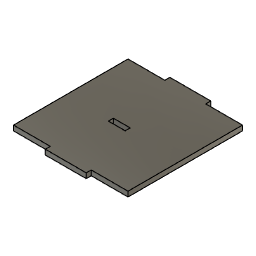
ProjectMiddle (Autodesk Fusion 360 design; units mm, degrees)
Autodesk Fusion 360 part; units mm, degrees
sketch "Sketch1" plane through (0, 0, 0) normal (0, 0, 1) x (1, 0, 0)
  line L0 (0, 0) -> (22, 0)
  line L1 (22, 0) -> (22, -3)
  line L2 (22, -3) -> (46.5, -3)
  line L3 (46.5, -3) -> (46.5, 0)
  line L4 (46.5, 0) -> (68.5, 0)
  line L5 (0, 0) -> (0, 68.5)
  line L6 (0, 68.5) -> (22, 68.5)
  line L7 (22, 68.5) -> (22, 71.5)
  line L8 (22, 71.5) -> (46.5, 71.5)
  line L9 (46.5, 71.5) -> (46.5, 68.5)
  line L10 (46.5, 68.5) -> (68.5, 68.5)
  line L11 (68.5, 68.5) -> (68.5, 0)
  line L12 (26.2767, 30.4485) -> (36.3506, 30.4485)
  line L13 (36.3506, 30.4485) -> (36.3506, 33.4485)
  line L14 (36.3506, 33.4485) -> (26.2767, 33.4485)
  line L15 (26.2767, 33.4485) -> (26.2767, 30.4485)
  dimension "d1" = 22
  dimension "d2" = 3
  dimension "d3" = 24.5
  dimension "d4" = 22
  dimension "d5" = 68.5
  dimension "d6" = 22
  dimension "d7" = 3
  dimension "d8" = 24.5
  dimension "d9" = 3
  dimension "d10" = 22
  dimension "d11" = 3
  constraint coincident L0.start L5.start
  constraint horizontal L0
  constraint perpendicular L0 L1
  constraint perpendicular L1 L2
  constraint perpendicular L2 L3
  constraint perpendicular L3 L4
  constraint vertical L5
  constraint perpendicular L5 L6
  constraint vertical L7
  constraint perpendicular L7 L8
  constraint vertical L9
  constraint perpendicular L9 L10
  constraint perpendicular L4 L11
  constraint horizontal L12
  constraint vertical L13
  constraint horizontal L14
  constraint vertical L15
  measures "d1" distance of L0.start L0.end
  measures "d2" distance of L0.end L1.end
  measures "d3" distance of L1.end L2.end
  measures "d4" distance of L3.end L4.end
  measures "d5" distance of L0.start L5.end
  measures "d6" distance of L5.end L6.end
  measures "d7" distance of L6.end L7.end
  measures "d8" distance of L7.end L8.end
  measures "d9" distance of L8.end L9.end
  measures "d10" distance of L9.end L10.end
  measures "d11" distance of L12.start L14.end
extrude "Extrude1" add sketch "Sketch1" along normal blind 3
